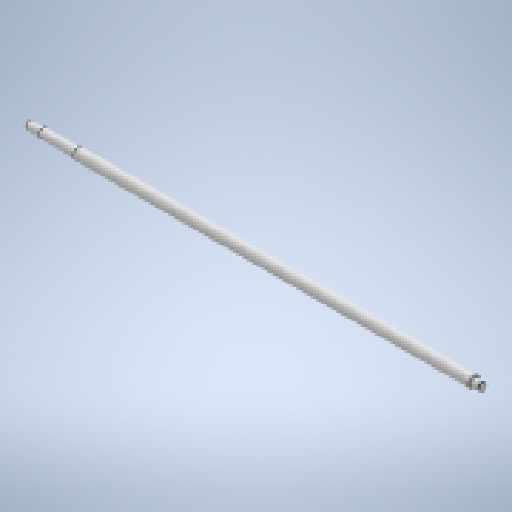
# Autodesk Inventor part: SFU1204-800
Saved by Autodesk Inventor 2023 (Build 270158000, 158)
## iProperties
Created: 2022-04-29
Part Number: SFU1204-800
Material: Generic
Document SubType Name: Modeling
Designer: plebbb
Density: 1 g/cm^3
Appearance: Default
Mass: 53.5524 g
Surface Area: 184.267 cm^2
Volume: 53.5524 cm^3
Author: plebbb
Autodesk Inventor part; units mm, degrees
ref_plane "YZ Plane" through (0, 0, 0) normal (1, 0, 0) x (0, 1, 0)
ref_plane "XZ Plane" through (0, 0, 0) normal (0, 1, 0) x (-1, 0, 0)
ref_plane "XY Plane" through (0, 0, 0) normal (0, 0, 1) x (1, 0, 0)
sketch "Sketch1" plane through (0, 0, 0) normal (0, 0, 1) x (1, 0, 0)
  line L0 (0, 4) -> (1, 4) construction
  line L1 (15, 4) -> (16, 5)
  line L2 (16, 5) -> (54, 5)
  line L3 (0, 4) -> (0, 3) construction
  line L4 (54, 5) -> (55, 6)
  line L5 (55, 6) -> (489, 6)
  line L6 (0, 3) -> (1, 4)
  line L7 (0, 3) -> (0, 0)
  line L8 (1, 4) -> (15, 4)
  line L9 (489, 6) -> (490, 5)
  line L10 (490, 5) -> (490, 4)
  line L11 (490, 4) -> (497, 4)
  line L12 (497, 4) -> (497, 3.8)
  line L13 (497, 3.8) -> (497.9, 3.8)
  line L14 (497.9, 3.8) -> (497.9, 4)
  line L15 (497.9, 4) -> (499, 4)
  line L16 (499, 4) -> (500, 3)
  line L17 (500, 3) -> (500, 0)
  line L18 (0, 0) -> (500, 0)
  point P0 (0, 0)
  point P1 (500, 1.5)
  dimension "d0" = 4
  dimension "d1" = 5
  dimension "d2" = 6
  dimension "d3" = 135
  dimension "d4" = 135
  dimension "d5" = 15
  dimension "d6" = 39
  dimension "d7" = 135
  dimension "d8" = 4
  dimension "d9" = 7
  dimension "d10" = 10
  dimension "d11" = 0.2
  dimension "d12" = 0.9
  dimension "d14" = 135
  dimension "d15" = 500
  constraints: 38 end point, 4 equal length, 4 horizontal, 4 perpendicular, 3 parallel, 3 vertical, 2 point on line, 1 coincident, 1 horizontal alignment, 1 midpoint
  measures "d0" distance of L0.start L7.end
  measures "d1" distance from line of L7.end L2
  measures "d2" distance from line of L7.end L5
  measures "d3" angle of L3 L6
  measures "d4" angle of L0 L1
  measures "d5" horizontal distance of L1.start point (0, 0)
  measures "d6" horizontal distance of L2.end L1.start
  measures "d7" angle of L9 L5
  measures "d8" distance from line of L17.end L15
  measures "d9" horizontal distance of L9.end L11.end
  measures "d10" horizontal distance of L9.end L16.end
  measures "d11" distance of L11.end L12.end
  measures "d12" distance of L12.end L13.end
  measures "d14" angle of L15 L16
  measures "d15" distance from line of point (500, 1.5) L7
revolve "Revolution1" add sketch "Sketch1" angle 360 about axis through (0, 0, 0) along (1, 0, 0)
equation "\"d15\" = SHAFT_LEN"
equation "\"SHAFT_LEN\" = 500"
body "Solid1"
